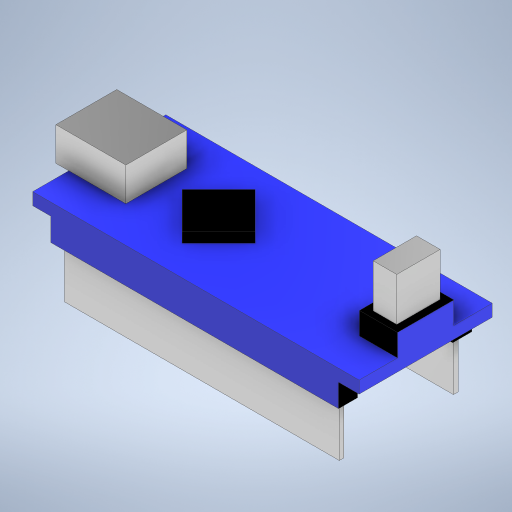
# Autodesk Inventor part: Arduino
Saved by Autodesk Inventor 2024 (Build 280153000, 153)
## iProperties
Created: 2024-05-29
Part Number: Arduino
Material: Genérico
Document SubType Name: Modeling
Designer: alexa
Density: 1 g/cm^3
Appearance: Valor por defecto
Author: alexa
Autodesk Inventor part; units mm, degrees
ref_plane "YZ Plane" through (0, 0, 0) normal (1, 0, 0) x (0, 1, 0)
ref_plane "XZ Plane" through (0, 0, 0) normal (0, 1, 0) x (-1, 0, 0)
sketch "Sketch1" plane through (0, 0, 0) normal (0, 1, 0) x (-1, 0, 0)
  line L0 (-21.45, 8.75) -> (21.45, 8.75)
  line L1 (21.45, 8.75) -> (21.45, -8.75)
  line L2 (21.45, -8.75) -> (-21.45, -8.75)
  line L3 (-21.45, -8.75) -> (-21.45, 8.75)
  line L4 (-21.45, 8.75) -> (21.45, -8.75) construction
  line L5 (21.45, 8.75) -> (-21.45, -8.75) construction
  point P0 (0, 0)
  dimension "d0" = 42.9
  dimension "d1" = 17.5
  constraints: 12 end point, 2 midpoint, 2 parallel, 1 horizontal, 1 perpendicular
  measures "d0" distance of L1.end L2.end
  measures "d1" distance of L0.end L1.end
extrude "Extrusion1" add sketch "Sketch1" along normal blind 1.6
sketch "Sketch2" plane through (0, 0, 0) normal (0, -1, 0) x (1, 0, 0)
  line L0 (21.45, -8.75) -> (-21.45, -8.75) projected
  line L1 (-21.45, -8.75) -> (-19.05, -8.75)
  line L2 (-19.05, -8.75) -> (18.75, -8.75)
  line L3 (18.75, -8.75) -> (18.75, -6.25)
  line L4 (18.75, -6.25) -> (-19.05, -6.25)
  line L5 (-19.05, -6.25) -> (-19.05, -8.75)
  point P0 (0, 0)
  dimension "d4" = 2.4
  dimension "d5" = 37.8
  dimension "d6" = 2.5
  constraints: 10 end point, 2 parallel, 1 horizontal, 1 perpendicular, 1 point on line
  measures "d4" distance of L0.end L1.end
  measures "d5" distance of L4.end L3.end
  measures "d6" distance of L3.end L2.end
extrude "Extrusion2" add sketch "Sketch2" along normal blind 3
ref_plane "Work Plane1" through (21.45, 1.6, 0) normal (0, 0, -1) x (-1, 0, 0)
sketch "Sketch3" plane through (0, -3, 0) normal (0, -1, 0) x (1, 0, 0)
  line L0 (18.75, -6.25) -> (-19.05, -6.25) projected
  line L1 (-19.05, -8.75) -> (18.75, -8.75) projected
  line L2 (18.75, -6.25) -> (-19.05, -8.75)
  line L3 (18.75, -8.75) -> (-19.05, -6.25)
  line L4 (-18.2, -7.2) -> (17.9, -7.2)
  line L5 (17.9, -7.2) -> (17.9, -7.8)
  line L6 (17.9, -7.8) -> (-18.2, -7.8)
  line L7 (-18.2, -7.8) -> (-18.2, -7.2)
  line L8 (-18.2, -7.2) -> (17.9, -7.8) construction
  line L9 (17.9, -7.2) -> (-18.2, -7.8) construction
  point P0 (0, 0)
  point P1 (-0.15, -7.5)
  dimension "d10" = 36.1
  dimension "d11" = 0.6
  constraints: 16 end point, 3 midpoint, 2 parallel, 1 horizontal, 1 perpendicular
  measures "d10" distance of L5.end L6.end
  measures "d11" distance of L4.end L5.end
extrude "Extrusion3" add sketch "Sketch3" along normal blind 6.8 contours L4 L5 L6 L3 L2 | L2 L3 L4 | L3 L2 L6 L7 L4 | L3 L6 L2
mirror "Mirror1" about plane through (21.45, 1.6, 0) normal (0, 0, -1) of "Extrusion3", "Extrusion2"
sketch "Sketch4" plane through (0, 1.6, 0) normal (0, 1, 0) x (1, 0, 0)
  line L0 (-21.45, 8.75) -> (-21.45, -8.75) projected
  line L1 (-10.5583, 0) -> (-5.75, 4.8083)
  line L2 (-5.75, 4.8083) -> (-0.9417, 0)
  line L3 (-0.9417, 0) -> (-5.75, -4.8083)
  line L4 (-5.75, -4.8083) -> (-10.5583, 0)
  point P0 (0, 0)
  point P1 (-5.75, 0)
  dimension "d15" = 6.8
  constraints: 8 end point, 9 other
  measures "d15" distance of L1.end L2.end
extrude "Extrusion4" add sketch "Sketch4" along normal blind 1.3
sketch "Sketch5" plane through (0, 1.6, 0) normal (0, 1, 0) x (1, 0, 0)
  line L0 (21.45, -8.75) -> (21.45, 8.75) projected
  line L1 (21.45, -3.7) -> (16.45, -3.7)
  line L2 (16.45, -3.7) -> (16.45, 3.7)
  line L3 (16.45, 3.7) -> (21.45, 3.7)
  line L4 (21.45, 3.7) -> (21.45, -3.7)
  line L5 (21.45, -3.7) -> (16.45, 3.7) construction
  line L6 (16.45, -3.7) -> (21.45, 3.7) construction
  point P0 (0, 0)
  dimension "d19" = 5
  dimension "d20" = 7.4
  constraints: 12 end point, 2 parallel, 1 horizontal, 1 perpendicular
  measures "d19" distance of L2.end L3.end
  measures "d20" distance of L1.end L2.end
extrude "Extrusion5" add sketch "Sketch5" along normal blind 2.9
sketch "Sketch6" plane through (0, 4.5, 0) normal (0, 1, 0) x (1, 0, 0)
  line L0 (16.45, -3.7) -> (21.45, -3.7) projected
  line L1 (21.45, -8.75) -> (21.45, 8.75) projected
  line L2 (21.45, 3.7) -> (16.45, 3.7) projected
  line L3 (20.5, -2.85) -> (17.4, -2.85)
  line L4 (17.4, -2.85) -> (17.4, 2.85)
  line L5 (17.4, 2.85) -> (20.5, 2.85)
  line L6 (20.5, 2.85) -> (20.5, -2.85)
  line L7 (20.5, -2.85) -> (17.4, 2.85) construction
  line L8 (17.4, -2.85) -> (20.5, 2.85) construction
  point P0 (0, 0)
  point P1 (18.95, 0)
  dimension "d23" = 3.1
  dimension "d24" = 5.7
  constraints: 12 end point, 2 midpoint, 2 parallel, 1 horizontal, 1 perpendicular
  measures "d23" distance of L4.end L5.end
  measures "d24" distance of L3.end L4.end
extrude "Extrusion6" add sketch "Sketch6" along normal blind 5.7
sketch "Sketch7" plane through (0, 1.6, 0) normal (0, 1, 0) x (1, 0, 0)
  line L0 (-21.45, 8.75) -> (-21.45, -8.75) projected
  line L1 (-13.95, 4) -> (-23.15, 4)
  line L2 (-23.15, 4) -> (-23.15, -4)
  line L3 (-23.15, -4) -> (-13.95, -4)
  line L4 (-13.95, -4) -> (-13.95, 4)
  point P0 (0, 0)
  dimension "d29" = 9.2
  dimension "d30" = 8
  constraints: 8 end point, 2 parallel, 1 horizontal, 1 perpendicular
  measures "d29" distance of L3.end L2.end
  measures "d30" distance of L2.end L1.end
extrude "Extrusion7" add sketch "Sketch7" along normal blind 4.4
body "Solid1"
